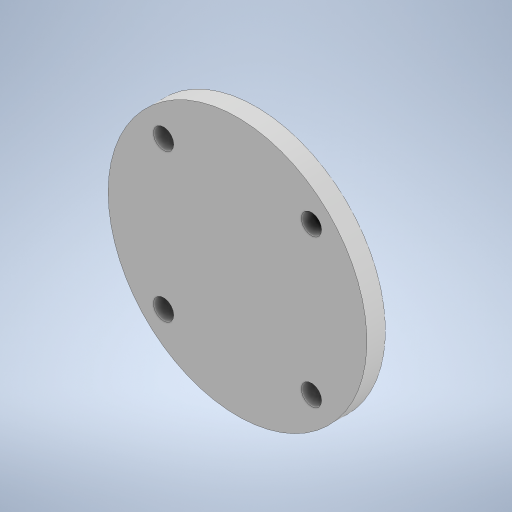
# Autodesk Inventor part: FlanschSchablone
Saved by Autodesk Inventor 2024.4 (Build 284460000, 460)
## iProperties
Created: 2025-12-03
Part Number: FlanschSchablone
Material: Generic
Document SubType Name: Modeling
Designer: jonas
Density: 1 g/cm^3
Appearance: Default
Author: jonas
Autodesk Inventor part; units mm, degrees
ref_plane "YZ Plane" through (0, 0, 0) normal (1, 0, 0) x (0, 1, 0)
ref_plane "XZ Plane" through (0, 0, 0) normal (0, 1, 0) x (-1, 0, 0)
ref_plane "XY Plane" through (0, 0, 0) normal (0, 0, 1) x (1, 0, 0)
sketch "Sketch1" plane through (0, 0, 0) normal (0, 1, 0) x (-1, 0, 0)
  circle A0 centre (0, 0) radius 35
  dimension "d0" = 70
  constraints: 1 centre point, 1 coincident
  measures "d0" diameter of A0
extrude "Extrusion1" add sketch "Sketch1" along normal blind 5
sketch "Sketch2" plane through (0, 5, 0) normal (0, 1, 0) x (1, 0, 0)
  circle A0 centre (0, 0) radius 7.5
  dimension "d3" = 15
  constraints: 1 centre point, 1 coincident
  measures "d3" diameter of A0
extrude "Extrusion2" add sketch "Sketch2" along normal blind 5
sketch "Sketch3" plane through (0, 0, 0) normal (0, -1, 0) x (1, 0, 0)
  line L0 (22.7941, 0) -> (-22.7941, 0) construction
  line L1 (0, 29.7059) -> (0, -29.7059) construction
  point P0 (0, 0)
  point P1 (20, 20)
  point P2 (20, -20)
  point P3 (-20, -20)
  point P4 (-20, 20)
  point P5 (0, 0)
  dimension "d6" = 40
  dimension "d7" = 40
  dimension "d8" = 20
  dimension "d9" = 20
  constraints: 4 end point, 2 horizontal alignment, 2 midpoint, 2 vertical alignment, 1 coincident, 1 horizontal, 1 vertical
  measures "d6" distance of point (-20, 20) point (20, 20)
  measures "d7" distance of point (20, -20) point (20, 20)
  measures "d8" distance from line of L0 point (20, 20)
  measures "d9" distance from line of L1 point (20, 20)
hole "Hole1" at (20, 0, 20) at (20, 0, -20) at (-20, 0, -20) at (-20, 0, 20) direction (0, 1, 0) diameter 5.5 end through all
body "Solid1"
